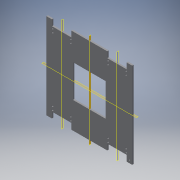
# Autodesk Inventor part: Milestone 8 & 9 Main Chasis
Saved by Autodesk Inventor 2016 (Build 200138000, 138)
## iProperties
Created: 2016-03-09
Part Number: Milestone 8 & 9 Main Chasis
Material: Generic
Document SubType Name: Modeling
Designer: Kenneth Daniel
Density: 1 g/cm^3
Appearance: Default
Mass: 634.326 g
Surface Area: 2169.18 cm^2
Volume: 634.326 cm^3
Author: Kenneth Daniel
Autodesk Inventor part; units mm, degrees
ref_plane "YZ Plane" through (0, 0, 0) normal (1, 0, 0) x (0, 1, 0)
ref_plane "XZ Plane" through (0, 0, 0) normal (0, 1, 0) x (-1, 0, 0)
ref_plane "XY Plane" through (0, 0, 0) normal (0, 0, 1) x (1, 0, 0)
sketch "Sketch1" plane through (0, 0, 0) normal (0, 1, 0) x (-1, 0, 0)
  line L0 (-175, 175) -> (-175, -175)
  line L1 (-175, -175) -> (175, -175)
  line L2 (175, -175) -> (175, 175)
  line L3 (175, 175) -> (-175, 175)
  line L4 (-175, 175) -> (175, -175) construction
  line L5 (-175, -175) -> (175, 175) construction
  line L6 (-86.5, 86.5) -> (86.5, 86.5)
  line L7 (86.5, 86.5) -> (86.5, -86.5)
  line L8 (86.5, -86.5) -> (-86.5, -86.5)
  line L9 (-86.5, -86.5) -> (-86.5, 86.5)
  line L10 (-86.5, 86.5) -> (86.5, -86.5) construction
  line L11 (86.5, 86.5) -> (-86.5, -86.5) construction
  line L12 (-66.5, 66.5) -> (-66.5, -66.5)
  line L13 (-66.5, -66.5) -> (66.5, -66.5)
  line L14 (66.5, -66.5) -> (66.5, 66.5)
  line L15 (66.5, 66.5) -> (-66.5, 66.5)
  line L16 (-66.5, 66.5) -> (66.5, -66.5) construction
  line L17 (-66.5, -66.5) -> (66.5, 66.5) construction
  line L18 (86.5, 0) -> (86.5, 20)
  line L19 (0, 233.3952) -> (0, -224.0457) construction
  line L20 (-86.5, -66.5) -> (-76.5, -66.5)
  line L21 (-76.5, -66.5) -> (-76.5, -76.5)
  line L22 (-76.5, -76.5) -> (-66.5, -76.5)
  line L23 (-66.5, -76.5) -> (-66.5, -86.5)
  line L24 (-66.5, 86.5) -> (-86.5, 86.5) construction
  line L25 (-86.5, 86.5) -> (-86.5, 66.5) construction
  line L26 (-86.5, 20) -> (-86.5, -20) construction
  line L27 (-86.5, -66.5) -> (-86.5, -86.5) construction
  line L28 (-86.5, -86.5) -> (-66.5, -86.5) construction
  point P0 (0, 0)
  dimension "d0" = 350
  dimension "d1" = 350
  dimension "d2" = 173
  dimension "d3" = 173
  dimension "d4" = 133
  dimension "d5" = 133
  constraints: 58 end point, 7 midpoint, 6 parallel, 5 collinear, 3 perpendicular, 3 vertical, 1 horizontal, 1 point on line, 1 symmetric about line
  measures "d0" distance of L0.start L0.end
  measures "d1" distance of L1.end L0.end
  measures "d2" distance of L6.start L6.end
  measures "d3" distance of L6.end L7.end
  measures "d4" distance of L12.start L12.end
  measures "d5" distance of L13.end L12.end
extrude "Extrusion1" add sketch "Sketch1" along normal blind 6.35 contours L3 L2 L1 L0 | L6 L7 L8 L23 L22 L21 L20 L9 | L20 L21 L22 L23 L8 L9
ref_plane "Work Plane1" through (0, 0, 175) normal (1, 0, 0) x (0, 0, -1)
mirror "Mirror1" about plane through (0, 0, 175) normal (1, 0, 0)
sketch "Sketch4" plane through (0, 0, 0) normal (0, -1, 0) x (1, 0, 0)
  line L0 (-175, -175) -> (-175, 175) projected
  line L1 (175, 175) -> (175, -175) projected
  line L2 (-175, 175) -> (175, -175) construction
  line L3 (175, -175) -> (-175, -175) projected
  line L4 (175, 175) -> (-175, -175) construction
  line L5 (-175, 97.632) -> (175, 97.632) construction
  line L6 (-175, 175) -> (175, 175) projected
  line L7 (-175, 175) -> (175, 175) projected
  line L8 (-147.197, 75.4377) -> (-147.197, 175)
  line L9 (-147.197, 75.4377) -> (-147.197, -175)
  point P0 (0, 0)
  point P1 (-140.5, -175)
  point P2 (-92.5, 175)
  point P3 (94.5, 175)
  point P4 (-140.5, 175)
  dimension "d43" = 77.368
  dimension "d46" = 27.803
  constraints: 10 end point, 5 point on line, 1 perpendicular
  measures "d43" distance between parallel lines of L5 L6
  measures "d46" distance between parallel lines of L0 L8
sketch "Sketch7" plane through (0, 6.35, 0) normal (0, 1, 0) x (1, 0, 0)
  line L0 (-175, 175) -> (-152, 175)
  line L1 (175, 175) -> (-175, 175) projected
  line L2 (-152, 175) -> (-73.5, 175)
  line L3 (-73.5, 175) -> (-73.5, 150.87)
  line L4 (-73.5, 150.87) -> (-152, 150.87)
  line L5 (-152, 150.87) -> (-152, 175)
  point P0 (0, 0)
  dimension "d55" = 23
  dimension "d56" = 78.5
  dimension "d58" = 24.13
  constraints: 10 end point, 2 perpendicular, 2 point on line, 1 vertical
  measures "d55" distance of L0.start L0.end
  measures "d56" distance of L0.end L2.end
  measures "d58" distance of L2.end L3.end
extrude "Extrusion6" cut sketch "Sketch7" against normal blind 10
mirror "Mirror6" about plane through (0, 0, 175) normal (1, 0, 0) of "Extrusion6", "Mirror1"
ref_plane "Work Plane5" through (-175, 0, 0) normal (0, 0, 1) x (1, 0, 0)
mirror "Mirror7" about plane through (-175, 0, 0) normal (0, 0, 1) of "Extrusion6", "Mirror1", "Mirror6"
ref_plane "Work Plane9" through (-112.75, 0, 150.87) normal (1, 0, 0) x (0, 0, -1)
sketch "Sketch9" plane through (0, 0, 0) normal (0, -1, 0) x (1, 0, 0)
  line L0 (73.5, 150.87) -> (152, 150.87) construction
  line L1 (112.75, 150.87) -> (112.75, 56.2031) construction
  line L2 (112.75, 150.87) -> (149.75, 150.87) construction
  line L3 (149.75, 150.87) -> (149.75, 18.2987) construction
  line L4 (149.75, 150.87) -> (149.75, 143.87) construction
  circle A0 centre (149.75, 143.87) radius 3.143
  line L5 (149.75, 143.87) -> (149.75, 129.87) construction
  circle A1 centre (149.75, 129.87) radius 3.143
  point P0 (0, 0)
  dimension "d76" = 37
  dimension "d77" = 7
  dimension "d78" = 6.286
  dimension "d79" = 14
  dimension "d80" = 6.286
  constraints: 10 end point, 3 point on line, 2 centre point, 2 coincident, 1 midpoint, 1 perpendicular, 1 vertical
  measures "d76" distance of L1.start L2.end
  measures "d77" distance of L2.end L4.end
  measures "d78" diameter of A0
  measures "d79" distance of L5.start L5.end
  measures "d80" diameter of A1
extrude "Extrusion8" cut sketch "Sketch9" against normal blind 10
ref_plane "Work Plane10" through (112.75, 0, 175) normal (-1, 0, 0) x (0, 0, 1)
mirror "Mirror10" about plane through (112.75, 0, 175) normal (-1, 0, 0) of "Extrusion8"
mirror "Mirror11" about plane through (0, 0, -175) normal (-1, 0, 0) of "Extrusion8", "Mirror10"
mirror "Mirror12" about plane through (-175, 0, 0) normal (0, 0, 1) of "Extrusion8", "Mirror10", "Mirror11"
sketch "Sketch10" plane through (0, 6.35, 0) normal (0, 1, 0) x (1, 0, 0)
  line L0 (152.0444, 151.0204) -> (175, 151.0204)
  line L1 (175, -175) -> (175, 175) projected
  line L2 (152, 175) -> (152, 150.87) projected
  line L3 (175, 151.0204) -> (152, 175)
  line L4 (175, 175) -> (152, 175) projected
  line L5 (152, 150.87) -> (175, 175)
  circle A0 centre (163.5, 162.935) radius 2.5
  point P0 (0, 0)
  dimension "d83" = 5
  constraints: 6 end point, 1 centre point, 1 horizontal, 1 midpoint, 1 point on line
  measures "d83" diameter of A0
extrude "Extrusion9" cut sketch "Sketch10" against normal through all contours A0 L3 L5 | L5 L3 A0 | L3 L5 A0 | L3 A0 L5
sketch "Sketch11" plane through (0, 0, 0) normal (0, -1, 0) x (1, 0, 0)
  line L0 (-90.2468, -110.8691) -> (-135.3673, -110.8691)
  line L1 (-135.3673, -110.8691) -> (-135.3673, -149.8508)
  line L2 (-135.3673, -149.8508) -> (-90.2468, -149.8508)
  line L3 (-90.2468, -149.8508) -> (-90.2468, -110.8691)
  circle A0 centre (-94.9188, -130.9693) radius 2.5175
  point P0 (0, 0)
  constraints: 8 end point, 2 parallel, 1 centre point, 1 horizontal, 1 perpendicular
extrude "Extrusion10" cut sketch "Sketch11" against normal blind 10 contours A0
mirror "Mirror13" about plane through (-112.75, 0, 150.87) normal (1, 0, 0) of "Extrusion10"
mirror "Mirror14" about plane through (-175, 0, 0) normal (0, 0, 1) of "Extrusion10", "Mirror13"
mirror "Mirror15" about plane through (0, 0, 175) normal (1, 0, 0) of "Extrusion10", "Mirror13", "Mirror14"
ref_plane "Work Plane2" through (0, 0, 175) normal (1, 0, 0) x (0, 0, -1)
ref_plane "Work Plane4" through (0, 0, 175) normal (1, 0, 0) x (0, 0, -1)
ref_plane "Work Plane6" through (0, 0, -175) normal (-1, 0, 0) x (0, 0, 1)
ref_plane "Work Plane7" through (0, 0, -175) normal (-1, 0, 0) x (0, 0, 1)
ref_plane "Work Plane8" through (0, 0, -175) normal (-1, 0, 0) x (0, 0, 1)
body "Solid1"
